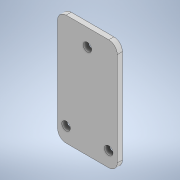
# Autodesk Inventor part: 6
Saved by Autodesk Inventor 2021 (Build 250183000, 183)
## iProperties
Created: 2021-03-30
Part Number: 6
Material: Genérico
Document SubType Name: Modeling
Designer: diego
Density: 1 g/cm^3
Appearance: Valor por defecto
Author: diego
Autodesk Inventor part; units mm, degrees
ref_plane "YZ Plane" through (0, 0, 0) normal (1, 0, 0) x (0, 1, 0)
ref_plane "XZ Plane" through (0, 0, 0) normal (0, 1, 0) x (-1, 0, 0)
ref_plane "XY Plane" through (0, 0, 0) normal (0, 0, 1) x (1, 0, 0)
sketch "Boceto1" plane through (0, 0, 0) normal (0, 0, 1) x (1, 0, 0)
  line L0 (5, 0) -> (30, 0)
  line L1 (35, 5) -> (35, 60)
  line L2 (30, 65) -> (5, 65)
  line L3 (0, 60) -> (0, 5)
  arc A0 (5, 65) -> (0, 60) centre (5, 60) ccw
  arc A1 (35, 60) -> (30, 65) centre (30, 60) ccw
  arc A2 (0, 5) -> (5, 0) centre (5, 5) ccw
  arc A3 (30, 0) -> (35, 5) centre (30, 5) ccw
  circle A4 centre (17.5, 55) radius 2.5
  circle A5 centre (5, 8.75) radius 2.5
  circle A6 centre (30, 8.75) radius 2.5
  point P0 (0, 0)
  constraints: 8 end point, 8 point on circle, 8 tangent, 7 centre point, 3 equal radius, 3 perpendicular, 2 point on line, 1 horizontal
extrude "Extrusión1" add sketch "Boceto1" along normal blind 3
